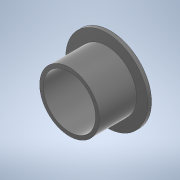
# Autodesk Inventor part: オイレスFd14D16L11
Saved by Autodesk Inventor 2020.2 (Build 242310000, 310)
## iProperties
Created: 2020-03-08
Part Number: オイレスFd14D16L11
Material: アセタール樹脂、黒
Document SubType Name: Modeling
Designer: aoyam
Density: 1.425 g/cm^3
Appearance: 滑らか - 黒
Mass: 0.285394 g
Surface Area: 4.79093 cm^2
Volume: 0.200277 cm^3
Author: aoyam
Autodesk Inventor part; units mm, degrees
ref_plane "YZ Plane" through (0, 0, 0) normal (1, 0, 0) x (0, 1, 0)
ref_plane "XZ Plane" through (0, 0, 0) normal (0, 1, 0) x (-1, 0, 0)
ref_plane "XY Plane" through (0, 0, 0) normal (0, 0, 1) x (1, 0, 0)
sketch "スケッチ1" plane through (0, 0, 0) normal (0, 0, 1) x (1, 0, 0)
  circle A0 centre (0, 0) radius 7
  circle A1 centre (0, 0) radius 8
  circle A2 centre (0, 0) radius 11
  dimension "d0" = 14
  dimension "d1" = 16
  dimension "d2" = 22
  constraints: 3 centre point, 3 coincident
  measures "d0" diameter of A0
  measures "d1" diameter of A1
  measures "d2" diameter of A2
extrude "押し出し1" add sketch "スケッチ1" against normal blind 1 contours A1 | A2
extrude "押し出し2" add sketch "スケッチ1" along normal blind 10 contours A1
